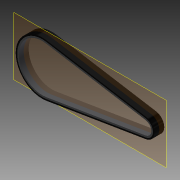
# Autodesk Inventor part: 285 mm Belt
Saved by Autodesk Inventor 2013 (Build 170138000, 138)
## iProperties
Created: 2013-06-27
Part Number: 285 mm Belt
Material: Generic
Document SubType Name: Modeling
Designer: mvarma
Density: 1 g/cm^3
Author: mvarma
Autodesk Inventor part; units mm, degrees
ref_plane "YZ Plane" through (0, 0, 0) normal (1, 0, 0) x (0, 1, 0)
ref_plane "XZ Plane" through (0, 0, 0) normal (0, 1, 0) x (-1, 0, 0)
ref_plane "XY Plane" through (0, 0, 0) normal (0, 0, 1) x (1, 0, 0)
sketch "Sketch1" plane through (0, 0, 0) normal (0, 0, 1) x (1, 0, 0)
  line L0 (3.7445, 22.5918) -> (94.5135, 7.547)
  line L1 (94.5135, -7.547) -> (3.7445, -22.5918)
  arc A0 (94.5135, -7.547) -> (94.5135, 7.547) centre (93.2626, 0) ccw
  arc A1 (3.7445, 22.5918) -> (3.7445, -22.5918) centre (0, 0) ccw
  line L2 (94.7211, 8.7999) -> (3.9522, 23.8447)
  arc A2 (3.9522, 23.8447) -> (3.9522, -23.8447) centre (0, 0) ccw
  line L3 (3.9522, -23.8447) -> (94.7211, -8.7999)
  arc A3 (94.7211, -8.7999) -> (94.7211, 8.7999) centre (93.2626, 0) ccw
  dimension "d7" = 1.27
  constraints: 8 end point, 8 point on circle, 4 centre point, 14 other
  measures "d7" distance between parallel lines of L2 L0
extrude "Extrusion1" add sketch "Sketch1" along normal blind 9
ref_plane "Work Plane1" through (0, 0, 4.5) normal (0, 0, 1) x (1, 0, 0)
sketch "Sketch2" plane through (0, 0, 4.5) normal (0, 0, 1) x (1, 0, 0)
  arc A0 (3.7445, 22.5918) -> (3.7445, -22.5918) centre (0, 0) ccw projected
  line L0 (94.5135, 7.547) -> (3.7445, 22.5918) projected
  arc A1 (94.5135, -7.547) -> (94.5135, 7.547) centre (93.2626, 0) ccw projected
  line L1 (3.7445, -22.5918) -> (94.5135, -7.547) projected
  arc A2 (3.4995, 21.1133) -> (3.4995, -21.1133) centre (0, 0) ccw
  line L2 (3.4995, 21.1133) -> (94.2684, 6.0686)
  arc A3 (94.2684, -6.0686) -> (94.2684, 6.0686) centre (93.2626, 0) ccw
  line L3 (94.2684, -6.0686) -> (3.4995, -21.1133)
  dimension "d11" = 1.4986
  constraints: 4 end point, 4 point on circle, 2 centre point, 3 other
  measures "d11" distance between parallel lines of L0 L2
extrude "Extrusion2" add sketch "Sketch2" along normal mid plane 8.9746
equation "\"d5\" = 45.8"
equation "\"d6\" = 15.3"
body "Solid1"
